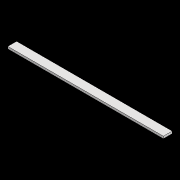
# Autodesk Inventor part: arm1_L
Saved by Autodesk Inventor 2022 (Build 260153000, 153)
## iProperties
Created: 2021-06-08
Part Number: arm1_L
Material: 一般
Document SubType Name: Modeling
Designer: yossy
Density: 1 g/cm^3
Appearance: 既定
Mass: 10.1259 g
Surface Area: 210.881 cm^2
Volume: 10.1259 cm^3
Author: yossy
Autodesk Inventor part; units mm, degrees
ref_plane "YZ Plane" through (0, 0, 0) normal (1, 0, 0) x (0, 1, 0)
ref_plane "XZ Plane" through (0, 0, 0) normal (0, 1, 0) x (-1, 0, 0)
ref_plane "XY Plane" through (0, 0, 0) normal (0, 0, 1) x (1, 0, 0)
sketch "スケッチ1" plane through (0, 0, 0) normal (0, 0, 1) x (1, 0, 0)
  line L0 (0, 0) -> (352, 0)
  line L1 (352, 0) -> (352, 5)
  line L2 (352, 5) -> (0, 5)
  line L3 (0, 5) -> (0, 0)
  line L4 (0, 0) -> (6, 0)
  line L5 (0, 1) -> (0, 0)
  dimension "d0" = 352
  dimension "d1" = 5
  constraints: 12 end point, 2 horizontal, 2 parallel, 1 perpendicular
  measures "d0" distance of L2.end L1.end
  measures "d1" distance of L1.end L0.end
extrude "押し出し1" add sketch "スケッチ1" along normal blind 20
sketch "スケッチ3" plane through (0, 0, 0) normal (-1, 0, 0) x (0, 0, 1)
  line L0 (0, 5) -> (0, 0) projected
  line L1 (0, 0) -> (20, 0) projected
  line L2 (20, 5) -> (20, 0) projected
  line L3 (0, 5) -> (20, 5) projected
  circle A0 centre (4, 2) radius 1.2
  circle A1 centre (16, 3) radius 1.2
  dimension "d14" = 2.4
  dimension "d15" = 2.4
  dimension "d16" = 3
  dimension "d17" = 4
  dimension "d18" = 4
  dimension "d19" = 3
  constraints: 2 centre point
  measures "d14" diameter of A0
  measures "d15" diameter of A1
  measures "d16" distance from line of L1 A1.centre
  measures "d17" distance from line of L2 A1.centre
  measures "d18" distance from line of L0 A0.centre
  measures "d19" distance from line of L3 A0.centre
extrude "押し出し3" cut sketch "スケッチ3" against normal blind 6 contours A0 | A1
sketch "スケッチ4" plane through (0, 0, 0) normal (0, -1, 0) x (1, 0, 0)
  line L0 (0, 0) -> (352, 0) projected
  line L1 (352, 0) -> (352, 20) projected
  line L2 (0, 20) -> (352, 20) projected
  line L3 (0, 0) -> (0, 20) projected
  line L4 (2, 2) -> (350, 2)
  line L5 (350, 2) -> (350, 18)
  line L6 (350, 18) -> (2, 18)
  line L7 (2, 18) -> (2, 2)
  dimension "d22" = 2
  dimension "d23" = 2
  dimension "d24" = 2
  dimension "d25" = 2
  constraints: 8 end point, 2 parallel, 1 horizontal, 1 perpendicular
  measures "d22" distance between parallel lines of L3 L7
  measures "d23" distance between parallel lines of L2 L6
  measures "d24" distance between parallel lines of L0 L4
  measures "d25" distance between parallel lines of L1 L5
extrude "押し出し4" cut sketch "スケッチ4" against normal blind 3 contours L7 L6 L5 L4
